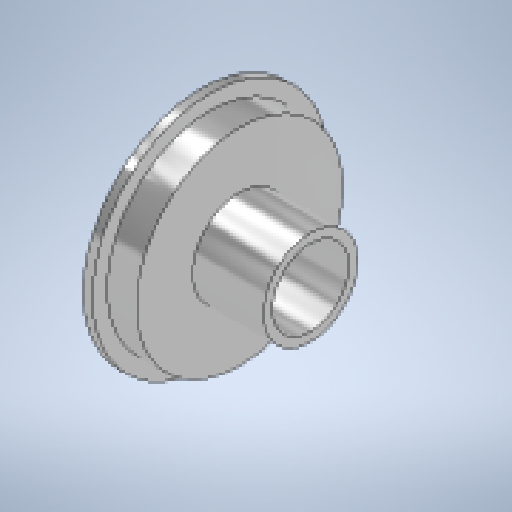
# Autodesk Inventor part: Base
Saved by Autodesk Inventor 2023.2 (Build 272271000, 271)
## iProperties
Created: 2024-01-10
Part Number: Base
Material: Aluminum 6061
Document SubType Name: Modeling
Designer: Nathan Cai
Density: 2.7 g/cm^3
Appearance: Aluminum - Flat
Author: Nathan Cai
Autodesk Inventor part; units mm, degrees
ref_plane "YZ Plane" through (0, 0, 0) normal (1, 0, 0) x (0, 1, 0)
ref_plane "XZ Plane" through (0, 0, 0) normal (0, 1, 0) x (-1, 0, 0)
ref_plane "XY Plane" through (0, 0, 0) normal (0, 0, 1) x (1, 0, 0)
sketch "Sketch1" plane through (0, 0, 0) normal (0, 0, 1) x (1, 0, 0)
  line L0 (0, 0) -> (5, 0)
  line L1 (5, 0) -> (5, 17.5)
  line L2 (5, 17.5) -> (0, 17.5)
  line L3 (0, 17.5) -> (0, 0)
  line L4 (5, 0) -> (17, 0)
  line L5 (17, 0) -> (17, 6.5)
  line L6 (17, 6.5) -> (5, 6.5)
  line L7 (5, 6.5) -> (5, 0)
  line L8 (0, 0) -> (-2, 0)
  line L9 (-2, 0) -> (-2, 20)
  line L10 (-2, 20) -> (0, 20)
  line L11 (0, 20) -> (0, 0)
  line L12 (-2, 0) -> (2.5, 0)
  line L13 (2.5, 0) -> (2.5, 9)
  line L14 (2.5, 9) -> (-2, 9)
  line L15 (-2, 9) -> (-2, 0)
  line L16 (2.5, 0) -> (3.5, 0)
  line L17 (3.5, 0) -> (3.5, 7.5)
  line L18 (3.5, 7.5) -> (2.5, 7.5)
  line L19 (2.5, 7.5) -> (2.5, 0)
  line L20 (17, 6.5) -> (5, 6.5)
  line L21 (5, 6.5) -> (5, 8)
  line L22 (5, 8) -> (17, 8)
  line L23 (17, 8) -> (17, 6.5)
  line L24 (-2, 0) -> (17, 0)
  line L25 (17, 0) -> (17, 6.5)
  line L26 (17, 6.5) -> (-2, 6.5)
  line L27 (-2, 6.5) -> (-2, 0)
  line L28 (5, 8) -> (7, 8)
  line L29 (7, 8) -> (7, 10)
  line L30 (7, 10) -> (5, 10)
  line L31 (5, 10) -> (5, 8)
  point P0 (-2, 9)
  point P1 (2.5, 7.5)
  point P2 (3.5, 6.5)
  point P3 (5, 6.5)
  dimension "d0" = 5
  dimension "d1" = 17.5
  dimension "d2" = 12
  dimension "d3" = 6.5
  dimension "d4" = 2
  dimension "d5" = 20
  dimension "d6" = 4.5
  dimension "d7" = 9
  dimension "d8" = 1
  dimension "d9" = 7.5
  dimension "d10" = 1.5
  dimension "d12" = 2
  dimension "d13" = 2
  constraints: 64 end point, 16 parallel, 8 horizontal, 8 perpendicular, 1 point on line
  measures "d0" distance of L2.end L1.end
  measures "d1" distance of L1.end L0.end
  measures "d2" distance of L6.end L5.end
  measures "d3" distance between parallel lines of L4 L6
  measures "d4" distance of L9.end L10.end
  measures "d5" distance between parallel lines of L8 L10
  measures "d6" distance of L14.end L13.end
  measures "d7" distance of L13.end L12.end
  measures "d8" distance of L18.end L17.end
  measures "d9" distance of L17.end L16.end
  measures "d10" distance of L20.end L21.end
  measures "d12" distance of L30.end L29.end
  measures "d13" distance of L29.end L28.end
revolve "Revolution1" add sketch "Sketch1" angle 360 about axis through (-2, 0, 0) along (1, 0, 0) contours L14 L9 L10 L11 L3 | L3 L2 L1 L26 L17 L18 L13 L14 | L1 L22 L23 L6 | L1 L30 L29 L22
sketch "Sketch2" plane through (5, 0, 0) normal (1, 0, 0) x (0, 0, -1)
  circle A0 centre (0, 0) radius 10 projected
  circle A1 centre (0, 0) radius 13.5 construction
  circle A2 centre (0, 13.5) radius 1.7526
  line L0 (0, 13.5) -> (0, 0) construction
  circle A3 centre (-11.6913, 6.75) radius 1.7526
  circle A4 centre (-11.6913, -6.75) radius 1.7526
  circle A5 centre (0, -13.5) radius 1.7526
  circle A6 centre (11.6913, -6.75) radius 1.7526
  circle A7 centre (11.6913, 6.75) radius 1.7526
  point P0 (0, 0)
  dimension "d14" = 27
  dimension "d15" = 3.5052
  dimension "d18" = 360
  constraints: 6 centre point, 2 end point, 1 coincident, 1 vertical, 1 vertical alignment, 15 other
  measures "d15" diameter of A2
extrude "Extrusion1" cut sketch "Sketch2" against normal through all contours A2 | A3 | A4 | A5 | A6 | A7
body "Solid1"
